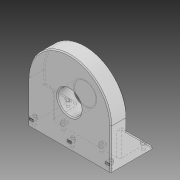
# Autodesk Inventor part: J0_drivebracket
Saved by Autodesk Inventor 2020 (Build 240168000, 168)
## iProperties
Created: 2021-03-20
Part Number: J0_drivebracket
Material: Generic
Document SubType Name: Modeling
Designer: DDeGo
Density: 1 g/cm^3
Appearance: Default
Author: DDeGo
Autodesk Inventor part; units mm, degrees
ref_plane "YZ Plane" through (0, 0, 0) normal (1, 0, 0) x (0, 1, 0)
ref_plane "XZ Plane" through (0, 0, 0) normal (0, 1, 0) x (-1, 0, 0)
ref_plane "XY Plane" through (0, 0, 0) normal (0, 0, 1) x (1, 0, 0)
sketch "Sketch1" plane through (0, 0, 0) normal (0, 0, 1) x (1, 0, 0)
  circle A0 centre (0, 0) radius 23.55
  arc A1 (82.55, 0) -> (-82.55, 0) centre (0, 0) ccw
  line L0 (-82.55, 0) -> (-82.55, -80)
  line L1 (-82.55, -80) -> (82.55, -80)
  line L2 (82.55, -80) -> (82.55, 0)
  dimension "d0" = 47.1
  dimension "d2" = 80
  dimension "d43" = 82.55
  constraints: 6 end point, 2 centre point, 2 coincident, 2 point on circle, 2 tangent, 2 vertical, 1 perpendicular
  measures "d0" diameter of A0
  measures "d2" distance from line of L1 point (0, 0)
  measures "d43" radius of A1
extrude "Extrusion1" add sketch "Sketch1" along normal blind 32.5
sketch "Sketch2" plane through (0, 0, 0) normal (0, 0, -1) x (-1, 0, 0)
  circle A0 centre (0, 0) radius 23.55 projected
  circle A1 centre (0, 0) radius 21.55
  dimension "d5" = 2
  constraints: 1 centre point, 1 coincident
  measures "d5" radial gap between concentric circles of A0 A1
extrude "Extrusion2" add sketch "Sketch2" against normal blind 1
sketch "Sketch7" plane through (-82.55, -80, 0) normal (-1, 0, 0) x (0, 0, 1)
  line L0 (0, 0) -> (32.5, 0) projected
  line L1 (0, 0) -> (-50, 0)
  line L2 (-50, 0) -> (-50, 5)
  line L3 (0, 80) -> (0, 0) projected
  line L4 (-50, 5) -> (0, 55)
  line L5 (0, 0) -> (0, 55)
  dimension "d32" = 50
  dimension "d33" = 5
  dimension "d34" = 135
  constraints: 8 end point, 2 parallel, 1 horizontal, 1 point on line
  measures "d32" distance of L0.start L1.end
  measures "d33" distance of L1.end L2.end
  measures "d34" angle of L2 L4
extrude "Extrusion7" add sketch "Sketch7" against normal blind 15
mirror "Mirror1" about plane through (0, 0, 0) normal (1, 0, 0) of "Extrusion7"
sketch "Sketch5" plane through (-82.55, -80, 0) normal (0, -1, 0) x (1, 0, 0)
  circle A0 centre (6.5, 26) radius 2.75
  circle A1 centre (158.6, 26) radius 2.75
  circle A2 centre (120.575, 6.5) radius 2.75
  circle A3 centre (44.525, 6.5) radius 2.75
  circle A4 centre (82.55, 26) radius 2.75
  line L0 (6.5, 26) -> (82.55, 26) construction
  line L1 (82.55, 26) -> (158.6, 26) construction
  line L2 (120.575, 6.5) -> (44.525, 6.5) construction
  line L3 (82.55, 26) -> (82.55, 6.5) construction
  line L4 (82.55, 6.5) -> (82.55, 0) construction
  line L5 (0, 0) -> (165.1, 0) construction
  line L6 (0, 32.5) -> (165.1, 32.5) construction
  line L7 (0, 0) -> (0, 32.5) construction
  line L8 (44.525, 26) -> (44.525, 6.5) construction
  line L9 (0, -50) -> (15, -50) construction
  line L10 (7.5, -50) -> (7.5, -40) construction
  line L11 (165.1, -50) -> (150.1, -50) construction
  line L12 (157.6, -50) -> (157.6, -40) construction
  line L13 (157.6, -40) -> (7.5, -40) construction
  circle A5 centre (7.5, -40) radius 2.75
  circle A6 centre (157.6, -40) radius 2.75
  dimension "d16" = 5.5
  dimension "d17" = 6.5
  dimension "d18" = 6.5
  dimension "d19" = 6.5
  dimension "d37" = 10
  dimension "d39" = 19.5
  constraints: 18 end point, 7 centre point, 6 equal radius, 5 vertical, 4 midpoint, 3 horizontal, 2 coincident, 1 collinear, 1 perpendicular
  measures "d16" diameter of A0
  measures "d17" distance between parallel lines of L5 L2
  measures "d18" distance between parallel lines of L6 L0
  measures "d19" distance from line of L7 L0.start
  measures "d37" distance of L10.start L10.end
  measures "d39" distance of L8.start L2.end
extrude "Extrusion4" cut sketch "Sketch5" against normal blind 18
ref_plane "Work Plane1" through (-82.55, -65, 0) normal (0, -1, 0) x (1, 0, 0)
sketch "Sketch6" plane through (-82.55, -65, 0) normal (0, -1, 0) x (1, 0, 0)
  circle A0 centre (158.6, 26) radius 2.75 projected
  circle A1 centre (82.55, 26) radius 2.75 projected
  circle A2 centre (44.525, 6.5) radius 2.75 projected
  line L0 (158.6, 30.7343) -> (162.7, 28.3671) construction
  line L1 (162.7, 28.3671) -> (162.7, 23.6329)
  line L2 (162.7, 23.6329) -> (158.6, 21.2657)
  line L3 (158.6, 21.2657) -> (154.5, 23.6329)
  line L4 (154.5, 23.6329) -> (154.5, 28.3671)
  line L5 (154.5, 28.3671) -> (158.6, 30.7343) construction
  line L6 (82.55, 30.7343) -> (86.65, 28.3671) construction
  line L7 (86.65, 28.3671) -> (86.65, 23.6329)
  line L8 (86.65, 23.6329) -> (82.55, 21.2657)
  line L9 (82.55, 21.2657) -> (78.45, 23.6329)
  line L10 (78.45, 23.6329) -> (78.45, 28.3671)
  line L11 (78.45, 28.3671) -> (82.55, 30.7343) construction
  circle A3 centre (44.525, 6.5) radius 2.75 projected
  line L12 (44.525, 1.7657) -> (40.425, 4.1329) construction
  line L13 (40.425, 4.1329) -> (40.425, 8.8671)
  line L14 (40.425, 8.8671) -> (44.525, 11.2343)
  line L15 (44.525, 11.2343) -> (48.625, 8.8671)
  line L16 (48.625, 8.8671) -> (48.625, 4.1329)
  line L17 (48.625, 4.1329) -> (44.525, 1.7657) construction
  circle A4 centre (120.575, 6.5) radius 2.75 projected
  line L18 (120.575, 1.7657) -> (116.475, 4.1329) construction
  line L19 (116.475, 4.1329) -> (116.475, 8.8671)
  line L20 (116.475, 8.8671) -> (120.575, 11.2343)
  line L21 (120.575, 11.2343) -> (124.675, 8.8671)
  line L22 (124.675, 8.8671) -> (124.675, 4.1329)
  line L23 (124.675, 4.1329) -> (120.575, 1.7657) construction
  circle A5 centre (6.5, 26) radius 2.75 projected
  line L24 (6.5, 21.2657) -> (2.4, 23.6329)
  line L25 (2.4, 23.6329) -> (2.4, 28.3671)
  line L26 (2.4, 28.3671) -> (6.5, 30.7343) construction
  line L27 (6.5, 30.7343) -> (10.6, 28.3671) construction
  line L28 (10.6, 28.3671) -> (10.6, 23.6329)
  line L29 (10.6, 23.6329) -> (6.5, 21.2657)
  line L30 (162.7, 28.3671) -> (162.7, 36.5137)
  line L31 (162.7, 36.5137) -> (154.5, 36.5137)
  line L32 (154.5, 36.5137) -> (154.5, 28.3671)
  line L33 (124.675, 4.1329) -> (124.675, -4.3085)
  line L34 (124.675, -4.3085) -> (116.475, -4.3085)
  line L35 (116.475, -4.3085) -> (116.475, 4.1329)
  line L36 (48.625, 4.1329) -> (48.625, -4.965)
  line L37 (48.625, -4.965) -> (40.425, -4.965)
  line L38 (40.425, -4.965) -> (40.425, 4.1329)
  line L39 (59, 1) -> (106.1, 1) projected
  line L40 (10.6, 28.3671) -> (10.6, 34.5607)
  line L41 (10.6, 34.5607) -> (2.4, 34.5607)
  line L42 (2.4, 34.5607) -> (2.4, 28.3671)
  circle A6 centre (157.6, -40) radius 2.75 projected
  circle A7 centre (157.6, -40) radius 2.75 projected
  circle A8 centre (7.5, -40) radius 2.75 projected
  line L43 (157.6, -44.7343) -> (153.5, -42.3671)
  line L44 (153.5, -42.3671) -> (153.5, -37.6329)
  line L45 (153.5, -37.6329) -> (157.6, -35.2657)
  line L46 (157.6, -35.2657) -> (161.7, -37.6329)
  line L47 (161.7, -37.6329) -> (161.7, -42.3671)
  line L48 (161.7, -42.3671) -> (157.6, -44.7343)
  line L49 (7.5, -44.7343) -> (3.4, -42.3671)
  line L50 (3.4, -42.3671) -> (3.4, -37.6329)
  line L51 (3.4, -37.6329) -> (7.5, -35.2657)
  line L52 (7.5, -35.2657) -> (11.6, -37.6329)
  line L53 (11.6, -37.6329) -> (11.6, -42.3671)
  line L54 (11.6, -42.3671) -> (7.5, -44.7343)
  line L55 (86.65, 28.3671) -> (86.65, 41.9185)
  line L56 (86.65, 41.9185) -> (78.45, 41.9185)
  line L57 (78.45, 41.9185) -> (78.45, 28.3671)
  point P0 (82.55, 0)
  point P1 (48.625, 1)
  point P2 (40.425, 1)
  point P3 (124.675, 1)
  point P4 (116.475, 1)
  dimension "d23" = 8.2
  constraints: 114 end point, 12 vertical, 7 coincident, 7 perpendicular, 6 equal length, 3 collinear, 91 other
  measures "d23" distance between parallel lines of L4 L1
extrude "Extrusion5" cut sketch "Sketch6" along normal blind 4.5
fillet "Fillet1" radius 2 1 edges at (-23.55, 0, 32.5)
chamfer "Chamfer1" distance 2 angle 45 10 edges at (0, 82.55, 32.5) (-82.55, -40, 32.5) (82.55, -40, 32.5) (0, 82.55, 0) (-82.55, -12.5, 0) (82.55, -12.5, 0) (-82.55, -50, -25) (-67.55, -50, -25) (67.55, -50, -25) (82.55, -50, -25)
fillet "Fillet2" radius 5 4 edges at (-67.55, -53.9142, 0) (67.55, -53.9142, 0) (75.05, -25, 0) (-75.05, -25, 0)
extrude "Extrusion8" cut sketch "Sketch6" against normal blind 4.5 contours A6 | A8 | L43 L44 L45 L46 L47 L48 | L49 L50 L51 L52 L53 L54
equation "\"d18\" = d17"
equation "\"d19\" = d17"
body "Solid1"
